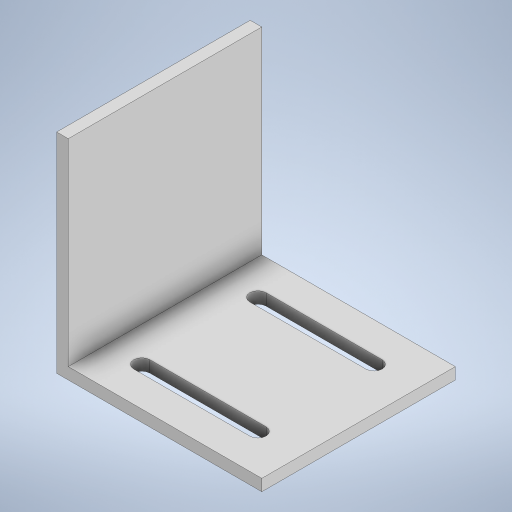
# Autodesk Inventor part: Nema 3 Mounting
Saved by Autodesk Inventor 2024 (Build 280153000, 153)
## iProperties
Created: 2024-01-25
Part Number: Nema 3 Mounting
Material: Generic
Document SubType Name: Modeling
Designer: aidan
Density: 1 g/cm^3
Appearance: Default
Author: aidan
Autodesk Inventor part; units mm, degrees
ref_plane "YZ Plane" through (0, 0, 0) normal (1, 0, 0) x (0, 1, 0)
ref_plane "XZ Plane" through (0, 0, 0) normal (0, 1, 0) x (-1, 0, 0)
ref_plane "XY Plane" through (0, 0, 0) normal (0, 0, 1) x (1, 0, 0)
sketch "Sketch1" plane through (0, 0, 0) normal (0, 1, 0) x (-1, 0, 0)
  line L0 (0, 0) -> (52.9999, 0)
  line L1 (52.9999, 0) -> (52.9999, 49.9999)
  line L2 (52.9999, 49.9999) -> (0, 49.9999)
  line L3 (0, 49.9999) -> (0, 0)
  dimension "d0" = 52.9999
  dimension "d1" = 49.9999
  constraints: 8 end point, 2 parallel, 1 horizontal, 1 perpendicular
  measures "d0" distance of L1.end L2.end
  measures "d1" distance of L0.end L1.end
extrude "Extrusion1" add sketch "Sketch1" along normal blind 3
sketch "Sketch2" plane through (0, 3, 0) normal (0, 1, 0) x (1, 0, 0)
  line L0 (-52.9999, 0) -> (-52.9999, -49.9999) projected
  line L1 (0, 0) -> (-52.9999, 0) projected
  line L2 (-52.9999, -49.9999) -> (-49.9999, -49.9999)
  line L3 (-49.9999, -49.9999) -> (-49.9999, 0)
  line L4 (-49.9999, 0) -> (-52.9999, 0)
  line L5 (-52.9999, 0) -> (-52.9999, -49.9999)
  dimension "d4" = 3
  constraints: 8 end point, 2 parallel, 1 horizontal, 1 perpendicular, 1 point on line
  measures "d4" distance of L0.end L2.end
extrude "Extrusion2" add sketch "Sketch2" along normal blind 50.9999
sketch "Sketch3" plane through (0, 3, 0) normal (0, 1, 0) x (1, 0, 0)
  line L0 (0, -49.9999) -> (0, 0) projected
  line L1 (0, -10.0051) -> (-11, -10.0051)
  circle A0 centre (-11, -10.0051) radius 2.1
  line L2 (-11, -10.0051) -> (-40.9999, -10.0051)
  circle A1 centre (-40.9999, -10.0051) radius 2.0955
  line L3 (-41.0003, -12.1006) -> (-11.0003, -12.1051)
  line L4 (-11.0003, -7.9051) -> (-41.0003, -7.9096)
  line L5 (0, -40.005) -> (-10.9982, -40.005)
  circle A2 centre (-10.9982, -40.005) radius 2.0955
  circle A3 centre (-41.0003, -40.005) radius 2.0955
  line L6 (-41.0003, -42.1005) -> (-10.9982, -42.1005)
  line L7 (-10.9982, -37.9095) -> (-41.0003, -37.9095)
  line L8 (-49.9999, -49.9999) -> (0, -49.9999) projected
  line L9 (0, 0) -> (-49.9999, 0) projected
  dimension "d7" = 11
  dimension "d8" = 4.2
  dimension "d9" = 29.9999
  dimension "d10" = 4.191
  dimension "d11" = 10.9982
  dimension "d12" = 4.191
  dimension "d13" = 4.191
  dimension "d14" = 29.9999
  dimension "d15" = 9.9949
  dimension "d16" = 10.0051
  constraints: 14 end point, 8 point on circle, 4 centre point, 3 coincident, 3 horizontal, 3 tangent, 2 point on line, 1 perpendicular
  measures "d7" distance of L1.start L1.end
  measures "d8" diameter of A0
  measures "d9" distance of L2.start L2.end
  measures "d10" diameter of A1
  measures "d11" distance of L5.start L5.end
  measures "d12" diameter of A2
  measures "d13" diameter of A3
  measures "d14" distance of L1.end L5.end
  measures "d15" distance between parallel lines of L8 L5
  measures "d16" distance between parallel lines of L9 L1
extrude "Extrusion3" cut sketch "Sketch3" against normal blind 12.5001
body "Solid1"
